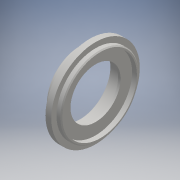
# Autodesk Inventor part: 2 крышка
Saved by Autodesk Inventor 2016 SP1 (Build 200210100, 210)
## iProperties
Created: 2016-05-01
Part Number: 2 крышка
Material: Типовые
Document SubType Name: Modeling
Designer: AS
Density: 1 g/cm^3
Appearance: По умолчанию
Author: AS
Autodesk Inventor part; units mm, degrees
ref_plane "YZ Plane" through (0, 0, 0) normal (1, 0, 0) x (0, 1, 0)
ref_plane "XZ Plane" through (0, 0, 0) normal (0, 1, 0) x (-1, 0, 0)
ref_plane "XY Plane" through (0, 0, 0) normal (0, 0, 1) x (1, 0, 0)
sketch "Эскиз1" plane through (0, 0, 0) normal (0, 0, 1) x (1, 0, 0)
  line L0 (-63.5, -92) -> (-63.5, -81)
  line L1 (-63.5, -81) -> (-63.5, -92)
  line L2 (-75.5, -92) -> (-75.5, -80)
  line L3 (-96.5, -62) -> (-68.5, -62)
  line L4 (-68.5, -62) -> (-68.5, -52)
  line L5 (-68.5, -52) -> (-63.5, -52)
  line L6 (-63.5, -52) -> (-63.5, -76)
  line L7 (-63.5, -76) -> (-53.5, -76)
  line L8 (-53.5, -76) -> (-53.5, -81)
  line L9 (-63.5, -92) -> (-75.5, -92)
  line L10 (-53.5, -81) -> (-63.5, -81)
  line L11 (-96.5, -70) -> (-90.5, -70)
  line L12 (-90.5, -70) -> (-75.5, -80)
  line L13 (-96.5, -62) -> (-96.5, -70)
  line L14 (-115.8, 0) -> (19.3, 0) projected
  point P0 (0, 0)
  dimension "d0" = 12
  dimension "d1" = 5
  dimension "d2" = 10
  dimension "d3" = 30
  dimension "d5" = 12
  dimension "d7" = 10
  dimension "d8" = 6
  dimension "d9" = 5
  dimension "d10" = 8
  dimension "d11" = 21
  dimension "d13" = 70
  constraints: 28 end point, 3 horizontal, 3 perpendicular, 2 point on line, 2 vertical, 1 collinear
  measures "d0" distance of L0.start L2.start
  measures "d1" distance of L7.end L8.end
  measures "d2" distance of L8.end L0.end
  measures "d3" distance between parallel lines of L3 L9
  measures "d5" distance of L2.start L2.end
  measures "d7" distance between parallel lines of L5 L3
  measures "d8" distance of L11.start L11.end
  measures "d9" distance between parallel lines of L4 L6
  measures "d10" distance between parallel lines of L3 L11
  measures "d11" horizontal distance of L11.start L2.start
  measures "d13" distance between parallel lines of L11 L14
revolve "Вращение1" add sketch "Эскиз1" angle 360 about axis through (-10, 0, 0) along (1, 0, 0)
chamfer "Фаска1" distance 2 angle 45 1 edges at (-96.5, 70, 0)
chamfer "Фаска2" distance 2 angle 45 1 edges at (-96.5, 62, 0)
chamfer "Фаска3" distance 2 angle 45 1 edges at (-53.5, 81, 0)
